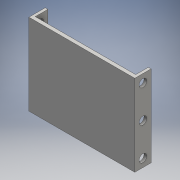
# Autodesk Inventor part: TrolleyBottomPlate
Saved by Autodesk Inventor 2016 (Build 200138000, 138)
## iProperties
Created: 2016-03-28
Part Number: TrolleyBottomPlate
Material: Generic
Document SubType Name: Modeling
Designer: mkepler
Density: 1 g/cm^3
Appearance: Default
Mass: 6.0793 g
Surface Area: 69.2832 cm^2
Volume: 6.0793 cm^3
Author: mkepler
Autodesk Inventor part; units mm, degrees
ref_plane "YZ Plane" through (0, 0, 0) normal (1, 0, 0) x (0, 1, 0)
ref_plane "XZ Plane" through (0, 0, 0) normal (0, 1, 0) x (-1, 0, 0)
ref_plane "XY Plane" through (0, 0, 0) normal (0, 0, 1) x (1, 0, 0)
sketch "Sketch1" plane through (0, 0, 0) normal (0, 1, 0) x (-1, 0, 0)
  line L0 (0, 0) -> (55.5, 0)
  line L1 (55.5, 0) -> (55.5, -45)
  line L2 (55.5, -45) -> (0, -45)
  line L3 (0, -45) -> (0, 0)
  dimension "d0" = 55.5
  dimension "d1" = 45
  constraints: 8 end point, 2 parallel, 1 horizontal, 1 perpendicular
  measures "d0" distance of L1.end L2.end
  measures "d1" distance of L0.end L1.end
extrude "Extrusion1" add sketch "Sketch1" along normal blind 2
sketch "Sketch2" plane through (0, 0, 0) normal (0, -1, 0) x (1, 0, 0)
  line L0 (0, -45) -> (-55.5, -45) projected
  line L1 (-55.5, -45) -> (-57, -45)
  line L2 (-57, -45) -> (-57, 0)
  line L3 (-57, 0) -> (-55.5, 0)
  line L4 (-55.5, 0) -> (-55.5, -45)
  line L5 (0, 0) -> (0, -45) projected
  line L6 (0, -45) -> (1.5, -45)
  line L7 (1.5, -45) -> (1.5, 0)
  line L8 (1.5, 0) -> (0, 0)
  line L9 (0, 0) -> (0, -45)
  dimension "d4" = 1.5
  dimension "d5" = 1.5
  constraints: 16 end point, 4 parallel, 2 horizontal, 2 perpendicular, 1 point on line
  measures "d4" distance of L2.end L3.end
  measures "d5" distance of L8.end L7.end
extrude "Extrusion2" add sketch "Sketch2" against normal blind 9
sketch "Sketch3" plane through (1.5, 0, 0) normal (1, 0, 0) x (0, 0, -1)
  circle A0 centre (4.5, 4.5) radius 2.15
  line L0 (45, 0) -> (0, 0) projected
  line L1 (0, 0) -> (0, 9) projected
  circle A1 centre (40.5, 4.5) radius 2.15
  line L2 (45, 0) -> (45, 9) projected
  circle A2 centre (22.5, 4.5) radius 2.15
  dimension "d8" = 4.3
  dimension "d9" = 4.5
  dimension "d10" = 4.5
  dimension "d11" = 4.3
  dimension "d12" = 4.5
  dimension "d13" = 4.5
  dimension "d14" = 4.3
  constraints: 3 centre point
  measures "d8" diameter of A0
  measures "d9" distance from line of A0.centre L0
  measures "d10" distance from line of L1 A0.centre
  measures "d11" diameter of A1
  measures "d12" distance from line of A1.centre L2
  measures "d13" distance from line of L0 A1.centre
  measures "d14" diameter of A2
hole "Hole1" at (1.5, 4.5, -4.5) at (1.5, 4.5, -22.5) at (1.5, 4.5, -40.5) direction (-1, 0, 0) diameter 4.3 end through all
body "Solid1"
